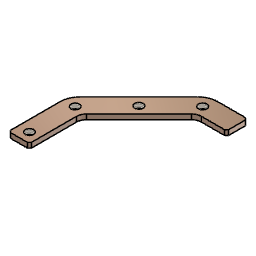
stage 2 shield 2 clamps v5 (Autodesk Fusion 360 design; units mm, degrees)
Autodesk Fusion 360 part; units mm, degrees
note: some values were not read from the file. Set by a fixed rule: which sketch regions a step uses; the direction of a hole.
sketch "Sketch1" plane through (0, 0, 0) normal (0, 1, 0) x (1, 0, 0)
  circle A0 centre (0, 0) radius 55 construction
  line L0 (48, 0) -> (48, 19.8823)
  line L1 (48, 19.8823) -> (19.8823, 48)
  line L2 (19.8823, 48) -> (-19.8823, 48)
  line L3 (-19.8823, 48) -> (-48, 19.8823)
  line L4 (-48, 19.8823) -> (-48, 0)
  line L5 (-48, 0) -> (48, 0) construction
  line L6 (0, -1.75) -> (0, -22.5) construction
  line L7 (50, 0) -> (50, 20.7107)
  line L8 (50, 20.7107) -> (20.7107, 50)
  line L9 (20.7107, 50) -> (-20.7107, 50)
  line L10 (-20.7107, 50) -> (-50, 20.7107)
  line L11 (-50, 20.7107) -> (-50, 0)
  line L12 (0, 0) -> (-54.6194, 22.6241) construction
  line L13 (60.5, 0) -> (60.5, 25.0599)
  line L14 (60.5, 25.0599) -> (25.0599, 60.5)
  line L15 (25.0599, 60.5) -> (-25.0599, 60.5)
  line L16 (-25.0599, 60.5) -> (-60.5, 25.0599)
  line L17 (-60.5, 25.0599) -> (-60.5, 0)
  line L18 (0, 60.5) -> (0, 50)
  line L19 (-50, 0) -> (-50, -5)
  line L20 (-50, -5) -> (-60.5, -5)
  line L21 (-60.5, -5) -> (-60.5, 0)
  line L22 (-6, 60.5) -> (-6, 50)
  point P0 (-55, 0)
  point P1 (-38.8909, -38.8909)
  point P2 (-54.6194, -22.6241)
  point P3 (0, -55)
  point P4 (-22.6241, -54.6194)
  point P5 (38.8909, -38.8909)
  point P6 (22.6241, -54.6194)
  point P7 (55, 0)
  point P8 (54.6194, -22.6241)
  point P9 (38.8909, 38.8909)
  point P10 (54.6194, 22.6241)
  point P11 (0, 55)
  point P12 (22.6241, 54.6194)
  point P13 (-38.8909, 38.8909)
  point P14 (-22.6241, 54.6194)
  dimension "d1" = 110
  dimension "d21" = 96
  dimension "d22" = 48
  dimension "d23" = 45
  dimension "d26" = 2
  dimension "d28" = 5
  dimension "d29" = 12.5
  dimension "d31" = 360
  dimension "d39" = 5
  dimension "d40" = 6
  constraint coincident A0.centre L12.start
  constraint horizontal L2
  constraint coincident A0 P0
  constraint horizontal A0.centre P0
  constraint equal L2 L3
  constraint equal L1 L2
  constraint equal L0 L4
  constraint horizontal L5
  constraint coincident A0.centre L5
  constraint coincident L3.end L12
  constraint coincident L15 L18.start
  constraint coincident L9 L18.end
  constraint perpendicular L9 L18
  constraint coincident P11 L18
  constraint parallel L11 L19
  constraint perpendicular L19 L20
  constraint collinear L17 L21
  measures "d1" diameter of A0
  measures "d21" distance of L0 L4
  measures "d22" distance of A0.centre L2
  measures "d23" angle of L2 L3
  measures "d28" distance of L10.end L12.end
  measures "d39" distance of P0 L20
extrude "Extrude3" add sketch "Sketch1" along normal blind 2.5 contours L9 L10 L11 L15 L16 L17 L19 L20 L21 L22
hole "Hole2" at (-54.6194, 0, -22.6241) at (-38.8909, 0, -38.8909) at (-22.6241, 0, -54.6194) at (-55, 0, 0) direction (0, 1, 0) diameter 4.234 depth 5 tip angle 118
thread "Thread1" "ISO Metric profile 5.0 M5x0.8 6H" thread offset 0 thread depth 10
fillet "Fillet1" radius 10 2 edges at (-60.5, 1.25, -25.0599) (-25.0599, 1.25, -60.5)
fillet "Fillet2" radius 5 2 edges at (-50, 1.25, -20.7107) (-20.7107, 1.25, -50)
chamfer "Chamfer2" distance 1 angle 45 4 edges at (-50, 1.25, 5) (-60.5, 1.25, 5) (-6, 1.25, -50) (-6, 1.25, -60.5)
sketch "stage 2 shield clamps cutting pattern" plane through (0, 2.5, 0) normal (0, 1, 0) x (-1, 0, 0)
  line L0 (6, -59.5) -> (7, -60.5)
  line L1 (7, -60.5) -> (20.9178, -60.5)
  arc A0 (20.9178, -60.5) -> (27.9889, -57.5711) centre (20.9178, -50.5) ccw
  line L2 (27.9889, -57.5711) -> (57.5711, -27.9889)
  arc A1 (57.5711, -27.9889) -> (60.5, -20.9178) centre (50.5, -20.9178) ccw
  line L3 (60.5, -20.9178) -> (60.5, 4)
  line L4 (60.5, 4) -> (59.5, 5)
  line L5 (59.5, 5) -> (51, 5)
  line L6 (51, 5) -> (50, 4)
  line L7 (50, 4) -> (50, -18.6396)
  arc A2 (48.5355, -22.1751) -> (50, -18.6396) centre (45, -18.6396) ccw
  line L8 (48.5355, -22.1751) -> (22.1751, -48.5355)
  arc A3 (18.6396, -50) -> (22.1751, -48.5355) centre (18.6396, -45) ccw
  line L9 (18.6396, -50) -> (7, -50)
  line L10 (7, -50) -> (6, -51)
  line L11 (6, -51) -> (6, -59.5)
  circle A4 centre (22.6241, -54.6194) radius 2.117
  circle A5 centre (54.6194, -22.6241) radius 2.117
  circle A6 centre (38.8909, -38.8909) radius 2.117
  circle A7 centre (55, 0) radius 2.117
